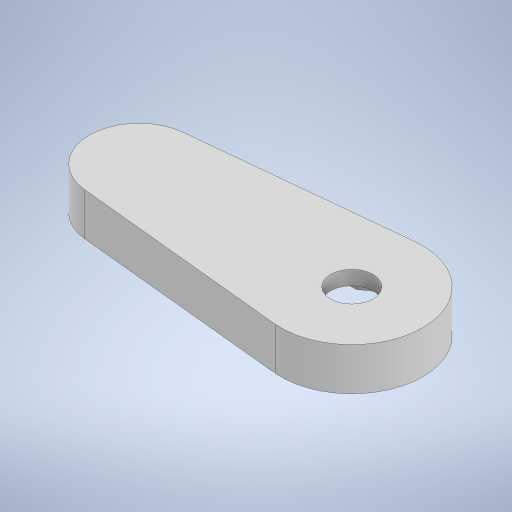
# Autodesk Inventor part: ServoAdapterB
Saved by Autodesk Inventor 2023.1 (Build 271208000, 208)
## iProperties
Created: 2023-04-23
Part Number: ServoAdapterB
Material: Generisch
Document SubType Name: Sheet Metal
Designer: marco
Density: 1 g/cm^3
Sheet Metal Rule: Standard_mm
Appearance: Vorgabe
Author: marco
Autodesk Inventor part; units mm, degrees
ref_plane "YZ Plane" through (0, 0, 0) normal (1, 0, 0) x (0, 1, 0)
ref_plane "XZ Plane" through (0, 0, 0) normal (0, 1, 0) x (-1, 0, 0)
ref_plane "XY Plane" through (0, 0, 0) normal (0, 0, 1) x (1, 0, 0)
sketch "Skizze1" plane through (0, 0, 0) normal (0, 1, 0) x (-1, 0, 0)
  circle A0 centre (0, 0) radius 1.5
  circle A1 centre (0, 0) radius 4
  circle A2 centre (0, 0) radius 5
  line L0 (12.9835, 1.4778) -> (12.9835, -5)
  circle A3 centre (15, 0) radius 2.5
  line L1 (2.6458, 3) -> (2.6458, -3)
  line L2 (15.1007, -2.498) -> (2.6458, -3)
  line L3 (15.1007, 2.498) -> (2.6458, 3)
  circle A4 centre (15, 0) radius 3.5
  line L4 (15.35, -3.4825) -> (0.5, -4.9749)
  line L5 (0.4089, 4.9832) -> (15.3498, 3.4825)
  dimension "d0" = 3
  dimension "d1" = 8
  dimension "d2" = 10
  dimension "d3" = 5
  dimension "d4" = 2.5
  dimension "d5" = 0
  dimension "d6" = 7
  dimension "d12" = 15
  constraints: 12 end point, 8 point on circle, 5 centre point, 5 tangent, 4 coincident, 2 vertical
  measures "d0" diameter of A0
  measures "d1" diameter of A1
  measures "d2" diameter of A2
  measures "d3" diameter of A3
  measures "d4" distance of A3.centre L0.start
  measures "d5" vertical distance of point (0, 0) A3.centre
  measures "d6" diameter of A4
  measures "d12" distance of A3.centre point (0, 0)
extrude "Extrusion1" add sketch "Skizze1" along normal blind 2 contours A1 L2 A2 L3 | A2 L5 A4 L3 | L2 A4 L0 L4 A2 | A4 L0 L2 A3 L3 | L2 L0 A4 | L0 A4 L4 picked at (-0.1239, 4.641) picked at (13.9331, -2.779)
sketch "Skizze2" plane through (-0.4089, 0, 4.9832) normal (-0.0999, 0, 0.995) x (0.995, 0, 0.0999)
  point P0 (-0.0912, 0)
sketch "Skizze3" plane through (0, 2, 0) normal (0, 1, 0) x (1, 0, 0)
  line L0 (-15.3498, -3.4825) -> (-0.4089, -4.9832) projected
  arc A0 (-0.4089, -4.9832) -> (-0.5, 4.9749) centre (0, 0) ccw projected
  arc A1 (-0.4089, -4.9832) -> (-0.5, 4.9749) centre (0, 0) ccw
  arc A2 (-15.35, 3.4825) -> (-15.3498, -3.4825) centre (-15, 0) ccw projected
  arc A3 (-15.35, 3.4825) -> (-15.3498, -3.4825) centre (-15, 0) ccw
  line L1 (-15.3498, -3.4825) -> (-0.4089, -4.9832)
  line L2 (-0.4089, -4.9832) -> (-0.5, 4.9749)
  line L3 (-0.5, 4.9749) -> (-15.35, 3.4825) projected
  line L4 (-15.35, 3.4825) -> (-0.5, 4.9749)
  circle A4 centre (0, 0) radius 1.5
  dimension "d9" = 3
  constraints: 6 end point, 4 point on circle, 3 centre point, 3 coincident, 1 collinear
  measures "d9" diameter of A4
extrude "Extrusion2" add sketch "Skizze3" along normal blind 1 contours A2 L3 L2 A4 L0 | L2 A4 A0
equation "\"Biegeradius\" = Stärke"
equation "\"BreiteBiegungsfreistellung\" = Stärke"
equation "\"TiefeBiegungsfreistellung\" = 0.5 * Stärke"
equation "\"GrößeEckenfreistellung\" = 4 * Stärke"
equation "\"MinimalRest\" = 2 * Stärke"
equation "\"Übergangsradius\" = Biegeradius"
equation "\"JacobiRadiusGröße\" = Biegeradius"
equation "\"Abstandsgröße\" = Stärke"
equation "\"Stärke\" = 0.5"
